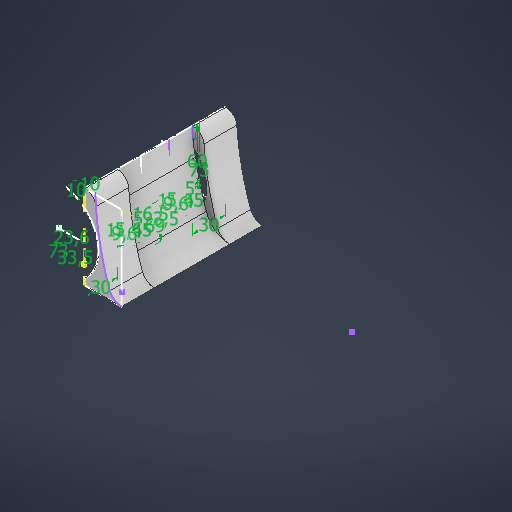
# Autodesk Inventor part: Ramp
Saved by Autodesk Inventor 2026.1 (Build 301233000, 233)
## iProperties
Created: 2026-05-18
Part Number: Ramp
Material: Generic
Document SubType Name: Modeling
Designer: 25adoh
Density: 1 g/cm^3
Appearance: Default
Author: 25adoh
Autodesk Inventor part; units mm, degrees
ref_plane "YZ Plane" through (0, 0, 0) normal (1, 0, 0) x (0, 1, 0)
ref_plane "XZ Plane" through (0, 0, 0) normal (0, 1, 0) x (-1, 0, 0)
ref_plane "XY Plane" through (0, 0, 0) normal (0, 0, 1) x (1, 0, 0)
sketch "Sketch1" plane through (0, 0, 0) normal (1, 0, 0) x (0, 1, 0)
  line L0 (0, -34.5) -> (0, 34.5)
  line L1 (0, 34.5) -> (9.6, 34.5)
  line L2 (9.6, 34.5) -> (9.6, 29.5)
  line L3 (9.6, 29.5) -> (0, 29.5)
  line L4 (0, 29.5) -> (0, 34.5)
  line L5 (0, 29.5) -> (4, 29.5)
  line L6 (4, 29.5) -> (4, 17.85)
  line L7 (4, 17.85) -> (0, 17.85)
  line L8 (0, 17.85) -> (0, 29.5)
  line L9 (0, 17.85) -> (10, 17.85)
  line L10 (10, 17.85) -> (10, 12.85)
  line L11 (10, 12.85) -> (0, 12.85)
  line L12 (0, 12.85) -> (0, 17.85)
  line L13 (9.6, 29.5) -> (4, 29.5)
  line L14 (4, 29.5) -> (4, 17.85)
  line L15 (4, 17.85) -> (9.6, 17.85)
  line L16 (9.6, 17.85) -> (9.6, 29.5)
  line L17 (0, -12.85) -> (9.6, -12.85)
  line L18 (9.6, -12.85) -> (9.6, -17.85)
  line L19 (9.6, -17.85) -> (0, -17.85)
  line L20 (0, -17.85) -> (0, -12.85)
  line L21 (0, -17.85) -> (4, -17.85)
  line L22 (4, -17.85) -> (4, -29.5)
  line L23 (4, -29.5) -> (0, -29.5)
  line L24 (0, -29.5) -> (0, -17.85)
  line L25 (0, -29.5) -> (10, -29.5)
  line L26 (10, -29.5) -> (10, -34.5)
  line L27 (10, -34.5) -> (0, -34.5)
  line L28 (0, -34.5) -> (0, -29.5)
  line L29 (9.6, -17.85) -> (4, -17.85)
  line L30 (4, -17.85) -> (4, -29.5)
  line L31 (4, -29.5) -> (9.6, -29.5)
  line L32 (9.6, -29.5) -> (9.6, -17.85)
  line L33 (0, 34.5) -> (60, 34.5)
  line L34 (60, 34.5) -> (60, -34.5)
  line L35 (60, -34.5) -> (0, -34.5)
  line L36 (0, -34.5) -> (0, 34.5)
  line L37 (0, 12.85) -> (60, 12.85)
  line L38 (60, 12.85) -> (60, -12.85)
  line L39 (60, -12.85) -> (0, -12.85)
  line L40 (0, -12.85) -> (0, 12.85)
  line L41 (0, 34.5) -> (0, -34.5)
  line L42 (0, -12.85) -> (0, 12.85)
  line L43 (0, 0) -> (16.5, 0)
  line L44 (16.5, 0) -> (-17, 0)
  line L45 (-17, -34.5) -> (-17, 34.5)
  line L46 (0, 34.5) -> (-17, 34.5)
  line L47 (-17, -34.5) -> (0, -34.5)
  line L48 (60, 34.5) -> (-17, 34.5)
  line L49 (-17, 34.5) -> (-17, 64.5)
  line L50 (-17, 64.5) -> (60, 64.5)
  line L51 (60, 64.5) -> (60, 34.5)
  line L52 (60, -34.5) -> (-17, -34.5)
  line L53 (-17, -34.5) -> (-17, -64.5)
  line L54 (-17, -64.5) -> (60, -64.5)
  line L55 (60, -64.5) -> (60, -34.5)
  dimension "d0" = 69
  dimension "d1" = 9.6
  dimension "d2" = 5
  dimension "d3" = 4
  dimension "d4" = 11.65
  dimension "d5" = 5
  dimension "d6" = 9.6
  dimension "d7" = 5
  dimension "d8" = 4
  dimension "d9" = 11.65
  dimension "d10" = 5
  dimension "d11" = 60
  dimension "d44" = 16.5
  dimension "d45" = 33.5
  dimension "d46" = 30
  dimension "d47" = 30
  constraints: 112 end point, 25 parallel, 14 horizontal, 12 perpendicular, 2 midpoint, 2 point on line, 1 collinear, 1 vertical
  measures "d0" distance of L0.start L0.end
  measures "d1" distance of L2.end L3.end
  measures "d2" distance of L1.end L2.end
  measures "d3" distance of L6.end L7.end
  measures "d4" distance of L5.end L6.end
  measures "d5" distance of L9.end L10.end
  measures "d6" distance of L29.start L21.start
  measures "d7" distance of L18.start L29.start
  measures "d8" distance of L22.end L23.end
  measures "d9" distance of L21.end L22.end
  measures "d10" distance of L25.end L27.start
  measures "d11" distance of L34.end L35.end
  measures "d44" distance of L43.start L43.end
  measures "d45" distance of L43.end L44.end
  measures "d46" distance of L48.end L49.end
  measures "d47" distance of L53.end L52.end
extrude "Extrusion1" add sketch "Sketch1" along normal blind 34
extrude "Extrusion2" add sketch "Sketch1" against normal blind 10 contours L22 L19 L32 L25 | L6 L3 L16 L9
sketch "Sketch7" plane through (0, -17, 64.5) normal (0, 0, 1) x (1, 0, 0)
  line L0 (0, 0) -> (0, 77) projected
  line L1 (0, 0) -> (34, 0)
  line L2 (34, 0) -> (34, 77)
  line L3 (34, 77) -> (0, 77)
  line L4 (0, 77) -> (0, 0)
  line L5 (0, 0) -> (0, 33.5)
  line L6 (0, 33.5) -> (-23.6, 33.5)
  circle A0 centre (-23.6, 33.5) radius 36.5
  line L7 (0, 77) -> (0, 67)
  line L8 (0, 77) -> (10, 77)
  arc A1 (23.1783, 7.1349) -> (34, 0) centre (34, 11.7743) ccw
  arc A2 (10, 77) -> (23.1783, 7.1349) centre (245.402, 85.2271) ccw
  point P0 (0, 17)
  dimension "d48" = 33.5
  dimension "d49" = 23.6
  dimension "d51" = 73
  dimension "d54" = 10
  dimension "d55" = 10
  constraints: 16 end point, 4 point on circle, 3 centre point, 3 point on line, 2 parallel, 2 perpendicular, 1 coincident, 1 horizontal, 1 tangent
  measures "d48" distance of L0.start L5.end
  measures "d49" distance of L5.end L6.end
  measures "d51" diameter of A0
  measures "d54" distance of L3.end L7.end
  measures "d55" distance of L3.end L8.end
extrude "Extrusion11" cut sketch "Sketch7" against normal up to surface (35 mm away) contours A0 L0 | L0 A0
extrude "Extrusion12" cut sketch "Sketch7" against normal up to surface (129 mm away) contours L3 L2 A1 A2
extrude "Extrusion13" add sketch "Sketch1" along normal blind 34 contours L47 L45 L44 L0 | L0 L23 L25 L26 L27 | L0 L19 L22 L23 | L26 L25 L32 L18 L39 L34 L35 | L0 L17 L18 L19 | L22 L19 L32 L25 | L45 L46 L0 L44 | L0 L11 L37 L34 L39 L17 | L37 L10 L9 L16 L2 L33 L34 | L0 L7 L9 L10 L11 | L1 L2 L3 L0 | L0 L3 L6 L7 | L6 L3 L16 L9
sketch "Sketch9" plane through (0, -17, -64.5) normal (0, 0, -1) x (-1, 0, 0)
  circle A0 centre (23.6, 33.5) radius 36.5
  point P0 (0, 17)
  dimension "d63" = 73
  constraints: 1 centre point, 1 coincident
  measures "d63" diameter of A0
extrude "Extrusion15" cut sketch "Sketch9" against normal up to surface (30 mm away)
sketch "Sketch8" plane through (10, 60, 34.5) normal (0, 0, 1) x (1, 0, 0)
  line L0 (0, 0) -> (24, 0) projected
  line L1 (-10, -71.344) -> (-10, -77) projected
  line L2 (24, 0) -> (-10, 0)
  line L3 (-10, 0) -> (-10, -77)
  line L4 (-10, -77) -> (24, -77)
  line L5 (24, -77) -> (24, 0)
  arc A0 (-10, 0) -> (24, -77) centre (94.1912, 0) ccw
  arc A1 (2.7208, -61.4849) -> (24, -77) centre (24, -54.6501) ccw
  arc A2 (-10, 0) -> (2.7208, -61.4849) centre (207.8306, 13.0094) ccw
  point P0 (-10, -60)
  point P1 (-7.3044, -23.5468)
  constraints: 8 end point, 7 point on circle, 3 centre point, 2 parallel, 2 tangent, 1 horizontal, 1 perpendicular
extrude "Extrusion14" cut sketch "Sketch8" against normal up to surface (69 mm away) contours L0 L5 A0 A2 L2 | A2 A0 | A1 A2 A0
fillet "Fillet1" radius 10 2 edges at (10, 60, 49.5) (10, 60, -49.5)
body "Solid1"
